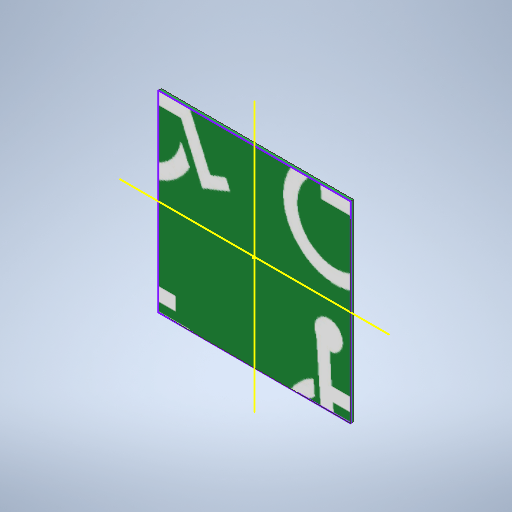
# Autodesk Inventor part: 비장애인
Saved by Autodesk Inventor 2025.1 (Build 291241000, 241)
## iProperties
Created: 2024-10-28
Part Number: 비장애인
Material: 장애인
Document SubType Name: Modeling
Designer: gmsee
Density: 1 g/cm^3
Appearance: 기본값(1)
Author: gmsee
Autodesk Inventor part; units mm, degrees
ref_plane "YZ Plane" through (0, 0, 0) normal (1, 0, 0) x (0, 1, 0)
ref_plane "XZ Plane" through (0, 0, 0) normal (0, 1, 0) x (-1, 0, 0)
ref_plane "XY Plane" through (0, 0, 0) normal (0, 0, 1) x (1, 0, 0)
sketch "스케치1" plane through (0, 0, 0) normal (0, 0, 1) x (1, 0, 0)
  line L0 (0, -89.6) -> (0, 89.6) projected
  line L1 (-89.6, 0) -> (89.6, 0) projected
  line L2 (-64, 64) -> (64, 64)
  line L3 (64, 64) -> (64, -64)
  line L4 (64, -64) -> (-64, -64)
  line L5 (-64, -64) -> (-64, 64)
  point P0 (0, 0)
  constraints: 8 end point, 2 parallel, 1 horizontal, 1 perpendicular
extrude "돌출1" add sketch "스케치1" against normal blind 2
